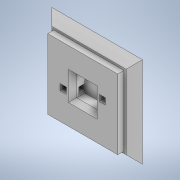
# Autodesk Inventor part: clear-square-reed
Saved by Autodesk Inventor 2021 (Build 250183000, 183)
## iProperties
Created: 2020-12-08
Part Number: clear-square-reed
Material: Generic
Document SubType Name: Modeling
Designer: Luke Kamols
Density: 1 g/cm^3
Appearance: Default
Author: Luke Kamols
Autodesk Inventor part; units mm, degrees
ref_plane "YZ Plane" through (0, 0, 0) normal (1, 0, 0) x (0, 1, 0)
ref_plane "XZ Plane" through (0, 0, 0) normal (0, 1, 0) x (-1, 0, 0)
ref_plane "XY Plane" through (0, 0, 0) normal (0, 0, 1) x (1, 0, 0)
sketch "Sketch1" plane through (0, 0, 0) normal (0, 0, 1) x (1, 0, 0)
  line L0 (0, 0) -> (44, 0)
  line L1 (44, 0) -> (44, 44)
  line L2 (44, 44) -> (0, 44)
  line L3 (0, 44) -> (0, 0)
  dimension "d0" = 44
  dimension "d1" = 44
  constraints: 8 end point, 2 parallel, 1 horizontal, 1 perpendicular
  measures "d0" distance of L2.end L1.end
  measures "d1" distance of L1.end L0.end
extrude "Extrusion1" add sketch "Sketch1" along normal blind 4
chamfer "Chamfer1" distance 4 angle 45 4 edges at (22, 44, 4) (44, 22, 4) (22, 0, 4) (0, 22, 4)
sketch "Sketch2" plane through (0, 0, 4) normal (0, 0, 1) x (1, 0, 0)
  line L0 (40, 4) -> (4, 4) projected
  line L1 (40, 40) -> (40, 4) projected
  line L2 (4, 40) -> (40, 40) projected
  line L3 (4, 4) -> (4, 40) projected
  line L4 (40, 4) -> (4, 4) projected
  line L5 (40, 40) -> (40, 4) projected
  line L6 (4, 4) -> (40, 40)
  line L7 (4, 40) -> (40, 40) projected
  line L8 (40, 4) -> (4, 40)
  line L9 (22, 27) -> (27, 27)
  line L10 (27, 27) -> (27, 17)
  line L11 (27, 17) -> (17, 17)
  line L12 (17, 27) -> (17, 17)
  line L13 (17, 27) -> (22, 27)
  point P0 (0, 0)
  constraints: 14 end point, 5 point on line, 4 perpendicular
extrude "Extrusion2" cut sketch "Sketch2" against normal blind 3 contours L11 L6 L8 | L8 L6 L10 | L12 L8 L6 | L6 L8 L13 L9
sketch "Sketch3" plane through (0, 0, 4) normal (0, 0, 1) x (1, 0, 0)
  line L0 (17, 27) -> (27, 27) projected
  line L1 (27, 27) -> (27, 17) projected
  line L2 (27, 17) -> (17, 17) projected
  line L3 (17, 17) -> (17, 27) projected
  line L4 (40, 4) -> (4, 4) projected
  line L5 (40, 40) -> (40, 4) projected
  line L6 (4, 40) -> (40, 40) projected
  line L7 (4, 4) -> (4, 40) projected
  line L8 (4, 4) -> (4, 40) projected
  line L9 (4, 4) -> (4, 5)
  line L10 (4, 5) -> (39, 5)
  line L11 (39, 5) -> (39, 39)
  line L12 (39, 39) -> (5, 39)
  line L13 (5, 39) -> (5, 5)
  point P0 (0, 0)
  dimension "d10" = 1
  dimension "d11" = 35
  dimension "d12" = 34
  dimension "d13" = 34
  constraints: 10 end point, 3 perpendicular, 2 point on line, 1 parallel
  measures "d10" distance of L4.end L9.end
  measures "d11" distance of L9.end L10.end
  measures "d12" distance of L10.end L11.end
  measures "d13" distance of L11.end L12.end
extrude "Extrusion3" add sketch "Sketch3" along normal blind 3 contours L13 L12 L11 L10
chamfer "Chamfer2" distance 2 angle 45 4 edges at (17, 22, 7) (22, 17, 7) (27, 22, 7) (22, 27, 7)
sketch "Sketch6" plane through (0, 0, 7) normal (0, 0, 1) x (1, 0, 0)
  line L0 (17, 27) -> (27, 27) projected
  line L1 (29, 15) -> (29, 29) projected
  line L2 (27, 27) -> (29, 27)
  line L3 (17, 17) -> (17, 27) projected
  line L4 (15, 29) -> (15, 15) projected
  line L5 (27, 17) -> (17, 17) projected
  line L6 (17, 17) -> (15, 17)
  line L7 (15, 17) -> (14, 17)
  line L8 (14, 17) -> (14, 18)
  line L9 (14, 18) -> (11, 18)
  line L10 (11, 18) -> (11, 21)
  line L11 (11, 21) -> (14, 21)
  line L12 (14, 21) -> (14, 18)
  line L13 (29, 27) -> (30, 27)
  line L14 (30, 27) -> (30, 26)
  line L15 (30, 26) -> (33, 26)
  line L16 (33, 26) -> (33, 23)
  line L17 (33, 23) -> (30, 23)
  line L18 (30, 23) -> (30, 26)
  point P0 (0, 0)
  dimension "d38" = 1
  dimension "d39" = 1
  dimension "d40" = 3
  dimension "d41" = 3
  dimension "d42" = 1
  dimension "d43" = 1
  dimension "d44" = 3
  dimension "d45" = 3
  constraints: 28 end point, 5 horizontal, 5 parallel, 4 perpendicular, 2 point on line
  measures "d38" distance of L6.end L7.end
  measures "d39" distance of L7.end L8.end
  measures "d40" distance of L10.end L11.end
  measures "d41" distance of L9.end L10.end
  measures "d42" distance of L2.end L13.end
  measures "d43" distance of L13.end L14.end
  measures "d44" distance of L16.end L17.end
  measures "d45" distance of L15.end L16.end
extrude "Extrusion4" cut sketch "Sketch6" against normal blind 5
sketch "Sketch7" plane through (27, 17, 1) normal (-1, 0, 0) x (0, 0, 1)
  line L0 (6, 9) -> (1, 9) projected
  line L1 (6, 6) -> (1, 6) projected
  line L2 (4, 10) -> (4, 0) projected
  line L3 (0, 10) -> (4, 10) projected
  line L4 (0, 10) -> (0, 0) projected
  line L5 (4, 0) -> (0, 0) projected
  line L6 (1, 9) -> (0, 9)
  line L7 (1, 6) -> (0, 6)
  line L8 (0, 10) -> (0, 0) projected
  line L9 (1, 6) -> (3, 6)
  line L10 (3, 6) -> (3, 9)
  point P0 (-1, -17)
  dimension "d48" = 2
  constraints: 8 end point, 4 point on line, 2 perpendicular, 1 horizontal
  measures "d48" distance of L1.end L9.end
extrude "Extrusion5" cut sketch "Sketch7" against normal blind 6 contours L10 L1 L7 L4 L6 L0
chamfer "Chamfer3" distance 1 angle 45 1 edges at (30, 24.5, 4)
chamfer "Chamfer4" distance 1 angle 45 1 edges at (33, 24.5, 1)
sketch "Sketch8" plane through (17, 17, 1) normal (1, 0, 0) x (0, 0, -1)
  line L0 (-6, 4) -> (-1, 4) projected
  line L1 (-6, 1) -> (-1, 1) projected
  line L2 (0, 0) -> (0, 10) projected
  line L3 (-1, 4) -> (0, 4)
  line L4 (-1, 1) -> (0, 1)
  line L5 (-1, 1) -> (-3, 1)
  line L6 (-3, 1) -> (-3, 4)
  point P0 (1, -17)
  dimension "d57" = 2
  constraints: 8 end point, 4 point on line, 2 perpendicular, 1 horizontal
  measures "d57" distance of L1.end L5.end
extrude "Extrusion6" cut sketch "Sketch8" against normal blind 6
chamfer "Chamfer5" distance 1 angle 45 2 edges at (11, 19.5, 1) (14, 19.5, 4)
body "Solid1"
